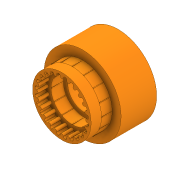
# Autodesk Inventor part: 4th Axis Barrel
Saved by Autodesk Inventor 2020 (Build 240168000, 168)
## iProperties
Created: 2021-06-26
Part Number: 4th Axis Barrel
Material: Generic
Document SubType Name: Modeling
Designer: Coy
Density: 1 g/cm^3
Appearance: Orange
Author: Coy
Autodesk Inventor part; units mm, degrees
ref_plane "YZ Plane" through (0, 0, 0) normal (1, 0, 0) x (0, 1, 0)
ref_plane "XZ Plane" through (0, 0, 0) normal (0, 1, 0) x (-1, 0, 0)
ref_plane "XY Plane" through (0, 0, 0) normal (0, 0, 1) x (1, 0, 0)
sketch "Sketch1" plane through (0, 0, 0) normal (0, 0, 1) x (1, 0, 0)
  circle A0 centre (0, 0) radius 11
  circle A1 centre (0, 0) radius 26
  dimension "d0" = 22
  dimension "d1" = 52
  constraints: 2 centre point, 2 coincident
  measures "d0" diameter of A0
  measures "d1" diameter of A1
extrude "Extrusion1" add sketch "Sketch1" against normal blind 24
sketch "Sketch2" plane through (0, 0, 0) normal (0, 0, 1) x (1, 0, 0)
  circle A0 centre (0, 0) radius 14
  circle A1 centre (0, 0) radius 20
  dimension "d4" = 28
  dimension "d5" = 40
  constraints: 2 centre point, 2 coincident
  measures "d4" diameter of A0
  measures "d5" diameter of A1
extrude "Extrusion2" add sketch "Sketch2" along normal blind 7
chamfer "Chamfer2" distance 7 angle 2 1 edges at (-20, 0, 7) measured on face at (-20, 0, 6.5)
sketch "Sketch4" plane through (0, 0, 7) normal (0, 0, 1) x (1, 0, 0)
  circle A0 centre (0, 0) radius 20 construction
  circle A1 centre (0, 0) radius 19.7556 projected
  arc A2 (0.2, 19.999) -> (-0.2, 19.999) centre (0, 20) ccw
  line L0 (-0.2, 19.999) -> (-0.1988, 19.7546)
  line L1 (0.2, 19.999) -> (0.1988, 19.7546)
  arc A3 (-7.4685, 18.5532) -> (-7.8381, 18.4001) centre (-7.6537, 18.4776) ccw
  line L2 (-7.8381, 18.4001) -> (-7.7434, 18.1748)
  line L3 (-7.4685, 18.5532) -> (-7.3761, 18.3269)
  arc A4 (-14, 14.2828) -> (-14.2828, 14) centre (-14.1421, 14.1421) ccw
  line L4 (-14.2828, 14) -> (-14.1091, 13.828)
  line L5 (-14, 14.2828) -> (-13.828, 14.1091)
  arc A5 (-18.4001, 7.8381) -> (-18.5532, 7.4685) centre (-18.4776, 7.6537) ccw
  line L6 (-18.5532, 7.4685) -> (-18.3269, 7.3761)
  line L7 (-18.4001, 7.8381) -> (-18.1748, 7.7434)
  arc A6 (-19.999, 0.2) -> (-19.999, -0.2) centre (-20, 0) ccw
  line L8 (-19.999, -0.2) -> (-19.7546, -0.1988)
  line L9 (-19.999, 0.2) -> (-19.7546, 0.1988)
  arc A7 (-18.5532, -7.4685) -> (-18.4001, -7.8381) centre (-18.4776, -7.6537) ccw
  line L10 (-18.4001, -7.8381) -> (-18.1748, -7.7434)
  line L11 (-18.5532, -7.4685) -> (-18.3269, -7.3761)
  arc A8 (-14.2828, -14) -> (-14, -14.2828) centre (-14.1421, -14.1421) ccw
  line L12 (-14, -14.2828) -> (-13.828, -14.1091)
  line L13 (-14.2828, -14) -> (-14.1091, -13.828)
  arc A9 (-7.8381, -18.4001) -> (-7.4685, -18.5532) centre (-7.6537, -18.4776) ccw
  line L14 (-7.4685, -18.5532) -> (-7.3761, -18.3269)
  line L15 (-7.8381, -18.4001) -> (-7.7434, -18.1748)
  arc A10 (-0.2, -19.999) -> (0.2, -19.999) centre (0, -20) ccw
  line L16 (0.2, -19.999) -> (0.1988, -19.7546)
  line L17 (-0.2, -19.999) -> (-0.1988, -19.7546)
  arc A11 (7.4685, -18.5532) -> (7.8381, -18.4001) centre (7.6537, -18.4776) ccw
  line L18 (7.8381, -18.4001) -> (7.7434, -18.1748)
  line L19 (7.4685, -18.5532) -> (7.3761, -18.3269)
  arc A12 (14, -14.2828) -> (14.2828, -14) centre (14.1421, -14.1421) ccw
  line L20 (14.2828, -14) -> (14.1091, -13.828)
  line L21 (14, -14.2828) -> (13.828, -14.1091)
  arc A13 (18.4001, -7.8381) -> (18.5532, -7.4685) centre (18.4776, -7.6537) ccw
  line L22 (18.5532, -7.4685) -> (18.3269, -7.3761)
  line L23 (18.4001, -7.8381) -> (18.1748, -7.7434)
  arc A14 (19.999, -0.2) -> (19.999, 0.2) centre (20, 0) ccw
  line L24 (19.999, 0.2) -> (19.7546, 0.1988)
  line L25 (19.999, -0.2) -> (19.7546, -0.1988)
  arc A15 (18.5532, 7.4685) -> (18.4001, 7.8381) centre (18.4776, 7.6537) ccw
  line L26 (18.4001, 7.8381) -> (18.1748, 7.7434)
  line L27 (18.5532, 7.4685) -> (18.3269, 7.3761)
  arc A16 (14.2828, 14) -> (14, 14.2828) centre (14.1421, 14.1421) ccw
  line L28 (14, 14.2828) -> (13.828, 14.1091)
  line L29 (14.2828, 14) -> (14.1091, 13.828)
  arc A17 (7.8381, 18.4001) -> (7.4685, 18.5532) centre (7.6537, 18.4776) ccw
  line L30 (7.4685, 18.5532) -> (7.3761, 18.3269)
  line L31 (7.8381, 18.4001) -> (7.7434, 18.1748)
  dimension "d25" = 0.4
  dimension "d28" = 360
  constraints: 64 end point, 35 point on circle, 16 centre point, 2 tangent, 132 other
  measures "d25" diameter of A2
extrude "Extrusion4" add sketch "Sketch4" against normal up to surface (7 mm away) contours A1 L24 A14 L25 | A1 L26 A15 L27 | L22 A13 L23 A1 | A1 L28 A16 L29 | L20 A12 L21 A1 | A1 L30 A17 L31 | L18 A11 L19 A1 | A1 L0 A2 L1 | L16 A10 L17 A1 | A1 L2 A3 L3 | L14 A9 L15 A1 | A1 L4 A4 L5 | L12 A8 L13 A1 | A1 L6 A5 L7 | L10 A7 L11 A1 | A1 L8 A6 L9
sketch "Sketch8" plane through (0, 0, 0) normal (0, 0, 1) x (1, 0, 0)
  circle A0 centre (0, 0) radius 14 projected
  circle A1 centre (0, 0) radius 11 projected
extrude "Extrusion7" cut sketch "Sketch8" against normal blind 1
chamfer "Chamfer4" distance 8 angle 2 1 edges at (-14, 0, 7) measured on face at (-14, 0, 6.5)
sketch "Sketch10" plane through (0, 0, 7) normal (0, 0, 1) x (1, 0, 0)
  circle A0 centre (0, 0) radius 14 construction
  circle A1 centre (0, 0) radius 14.2794 projected
  arc A2 (-0.2, 13.9986) -> (0.2, 13.9986) centre (0, 14) ccw
  line L0 (0.204, 14.2779) -> (0.2, 13.9971)
  line L1 (-0.204, 14.2779) -> (-0.2, 13.9971)
  line L2 (-7.3156, 12.263) -> (-7.1718, 12.0219)
  arc A3 (-7.1725, 12.0231) -> (-6.8261, 12.2231) centre (-7, 12.1244) ccw
  line L3 (-6.9623, 12.467) -> (-6.8254, 12.2219)
  line L4 (-12.467, 6.9623) -> (-12.2219, 6.8254)
  arc A4 (-12.2231, 6.8261) -> (-12.0231, 7.1725) centre (-12.1244, 7) ccw
  line L5 (-12.263, 7.3156) -> (-12.0219, 7.1718)
  line L6 (-14.2779, -0.204) -> (-13.9971, -0.2)
  arc A5 (-13.9986, -0.2) -> (-13.9986, 0.2) centre (-14, 0) ccw
  line L7 (-14.2779, 0.204) -> (-13.9971, 0.2)
  line L8 (-12.263, -7.3156) -> (-12.0219, -7.1718)
  arc A6 (-12.0231, -7.1725) -> (-12.2231, -6.8261) centre (-12.1244, -7) ccw
  line L9 (-12.467, -6.9623) -> (-12.2219, -6.8254)
  line L10 (-6.9623, -12.467) -> (-6.8254, -12.2219)
  arc A7 (-6.8261, -12.2231) -> (-7.1725, -12.0231) centre (-7, -12.1244) ccw
  line L11 (-7.3156, -12.263) -> (-7.1718, -12.0219)
  line L12 (0.204, -14.2779) -> (0.2, -13.9971)
  arc A8 (0.2, -13.9986) -> (-0.2, -13.9986) centre (0, -14) ccw
  line L13 (-0.204, -14.2779) -> (-0.2, -13.9971)
  line L14 (7.3156, -12.263) -> (7.1718, -12.0219)
  arc A9 (7.1725, -12.0231) -> (6.8261, -12.2231) centre (7, -12.1244) ccw
  line L15 (6.9623, -12.467) -> (6.8254, -12.2219)
  line L16 (12.467, -6.9623) -> (12.2219, -6.8254)
  arc A10 (12.2231, -6.8261) -> (12.0231, -7.1725) centre (12.1244, -7) ccw
  line L17 (12.263, -7.3156) -> (12.0219, -7.1718)
  line L18 (14.2779, 0.204) -> (13.9971, 0.2)
  arc A11 (13.9986, 0.2) -> (13.9986, -0.2) centre (14, 0) ccw
  line L19 (14.2779, -0.204) -> (13.9971, -0.2)
  line L20 (12.263, 7.3156) -> (12.0219, 7.1718)
  arc A12 (12.0231, 7.1725) -> (12.2231, 6.8261) centre (12.1244, 7) ccw
  line L21 (12.467, 6.9623) -> (12.2219, 6.8254)
  line L22 (6.9623, 12.467) -> (6.8254, 12.2219)
  arc A13 (6.8261, 12.2231) -> (7.1725, 12.0231) centre (7, 12.1244) ccw
  line L23 (7.3156, 12.263) -> (7.1718, 12.0219)
  point P0 (13.9986, -0.2)
  point P1 (12.0231, -7.1725)
  point P2 (6.8261, -12.2231)
  point P3 (-0.2, -13.9986)
  point P4 (-7.1725, -12.0231)
  point P5 (7.1725, 12.0231)
  point P6 (0.2, 13.9986)
  point P7 (-12.0231, 7.1725)
  point P8 (-13.9986, 0.2)
  dimension "d67" = 0.4
  dimension "d70" = 360
  constraints: 53 point on circle, 48 end point, 12 centre point, 2 line through centre, 2 tangent, 122 other
  measures "d67" diameter of A2
extrude "Extrusion8" add sketch "Sketch10" against normal up to surface (8 mm away) contours A1 L19 A11 L18 | L21 A12 L20 A1 | A1 L17 A10 L16 | L23 A13 L22 A1 | A1 L15 A9 L14 | L0 A2 L1 A1 | A1 L13 A8 L12 | L3 A3 L2 A1 | A1 L11 A7 L10 | L5 A4 L4 A1 | A1 L9 A6 L8 | L7 A5 L6 A1
sketch "Sketch12" plane through (0, 0, 7) normal (0, 0, 1) x (1, 0, 0)
  circle A0 centre (0, 0) radius 19.7556
  circle A1 centre (0, 0) radius 16.0556 construction
  line L0 (0, 0) -> (0, -27.6947) construction
  arc A2 (1.048, -17.0411) -> (-1.048, -17.0411) centre (0, -17.1056) ccw
  line L1 (-1.0542, -17.1411) -> (-1.048, -17.0411)
  line L2 (1.0542, -17.1411) -> (1.048, -17.0411)
  arc A3 (1.0542, -17.1411) -> (2.2305, -18.1188) centre (2.1022, -17.0766) ccw
  arc A4 (-2.2305, -18.1188) -> (-1.0542, -17.1411) centre (-2.1022, -17.0766) ccw
  arc A5 (5.4547, -16.2842) -> (6.844, -16.9241) centre (6.4503, -15.9507) ccw
  line L3 (5.4547, -16.2842) -> (5.4229, -16.1892)
  arc A6 (5.4229, -16.1892) -> (3.3983, -16.7317) centre (4.4272, -16.5227) ccw
  line L4 (3.4182, -16.8299) -> (3.3983, -16.7317)
  arc A7 (2.535, -18.0787) -> (3.4182, -16.8299) centre (2.3892, -17.0389) ccw
  arc A8 (9.4835, -14.3175) -> (10.991, -14.5761) centre (10.3589, -13.7377) ccw
  line L5 (9.4835, -14.3175) -> (9.4282, -14.234)
  arc A9 (9.4282, -14.234) -> (7.6129, -15.282) centre (8.5528, -14.8138) ccw
  line L6 (7.6576, -15.3717) -> (7.6129, -15.282)
  arc A10 (7.1277, -16.8066) -> (7.6576, -15.3717) centre (6.7178, -15.8399) ccw
  arc A11 (12.866, -11.3752) -> (14.3891, -11.2347) centre (13.5615, -10.5885) ccw
  line L7 (12.866, -11.3752) -> (12.7909, -11.3088)
  arc A12 (12.7909, -11.3088) -> (11.3088, -12.7909) centre (12.0955, -12.0955) ccw
  line L8 (11.3752, -12.866) -> (11.3088, -12.7909)
  arc A13 (11.2347, -14.3891) -> (11.3752, -12.866) centre (10.5885, -13.5615) ccw
  arc A14 (15.3717, -7.6576) -> (16.8066, -7.1277) centre (15.8399, -6.7178) ccw
  line L9 (15.3717, -7.6576) -> (15.282, -7.6129)
  arc A15 (15.282, -7.6129) -> (14.234, -9.4282) centre (14.8138, -8.5528) ccw
  line L10 (14.3175, -9.4835) -> (14.234, -9.4282)
  arc A16 (14.5761, -10.991) -> (14.3175, -9.4835) centre (13.7377, -10.3589) ccw
  arc A17 (16.8299, -3.4182) -> (18.0787, -2.535) centre (17.0389, -2.3892) ccw
  line L11 (16.8299, -3.4182) -> (16.7317, -3.3983)
  arc A18 (16.7317, -3.3983) -> (16.1892, -5.4229) centre (16.5227, -4.4272) ccw
  line L12 (16.2842, -5.4547) -> (16.1892, -5.4229)
  arc A19 (16.9241, -6.844) -> (16.2842, -5.4547) centre (15.9507, -6.4503) ccw
  arc A20 (17.1411, 1.0542) -> (18.1188, 2.2305) centre (17.0766, 2.1022) ccw
  line L13 (17.1411, 1.0542) -> (17.0411, 1.048)
  arc A21 (17.0411, 1.048) -> (17.0411, -1.048) centre (17.1056, 0) ccw
  line L14 (17.1411, -1.0542) -> (17.0411, -1.048)
  arc A22 (18.1188, -2.2305) -> (17.1411, -1.0542) centre (17.0766, -2.1022) ccw
  arc A23 (16.2842, 5.4547) -> (16.9241, 6.844) centre (15.9507, 6.4503) ccw
  line L15 (16.2842, 5.4547) -> (16.1892, 5.4229)
  arc A24 (16.1892, 5.4229) -> (16.7317, 3.3983) centre (16.5227, 4.4272) ccw
  line L16 (16.8299, 3.4182) -> (16.7317, 3.3983)
  arc A25 (18.0787, 2.535) -> (16.8299, 3.4182) centre (17.0389, 2.3892) ccw
  arc A26 (14.3175, 9.4835) -> (14.5761, 10.991) centre (13.7377, 10.3589) ccw
  line L17 (14.3175, 9.4835) -> (14.234, 9.4282)
  arc A27 (14.234, 9.4282) -> (15.282, 7.6129) centre (14.8138, 8.5528) ccw
  line L18 (15.3717, 7.6576) -> (15.282, 7.6129)
  arc A28 (16.8066, 7.1277) -> (15.3717, 7.6576) centre (15.8399, 6.7178) ccw
  arc A29 (11.3752, 12.866) -> (11.2347, 14.3891) centre (10.5885, 13.5615) ccw
  line L19 (11.3752, 12.866) -> (11.3088, 12.7909)
  arc A30 (11.3088, 12.7909) -> (12.7909, 11.3088) centre (12.0955, 12.0955) ccw
  line L20 (12.866, 11.3752) -> (12.7909, 11.3088)
  arc A31 (14.3891, 11.2347) -> (12.866, 11.3752) centre (13.5615, 10.5885) ccw
  arc A32 (7.6576, 15.3717) -> (7.1277, 16.8066) centre (6.7178, 15.8399) ccw
  line L21 (7.6576, 15.3717) -> (7.6129, 15.282)
  arc A33 (7.6129, 15.282) -> (9.4282, 14.234) centre (8.5528, 14.8138) ccw
  line L22 (9.4835, 14.3175) -> (9.4282, 14.234)
  arc A34 (10.991, 14.5761) -> (9.4835, 14.3175) centre (10.3589, 13.7377) ccw
  arc A35 (3.4182, 16.8299) -> (2.535, 18.0787) centre (2.3892, 17.0389) ccw
  line L23 (3.4182, 16.8299) -> (3.3983, 16.7317)
  arc A36 (3.3983, 16.7317) -> (5.4229, 16.1892) centre (4.4272, 16.5227) ccw
  line L24 (5.4547, 16.2842) -> (5.4229, 16.1892)
  arc A37 (6.844, 16.9241) -> (5.4547, 16.2842) centre (6.4503, 15.9507) ccw
  arc A38 (-1.0542, 17.1411) -> (-2.2305, 18.1188) centre (-2.1022, 17.0766) ccw
  line L25 (-1.0542, 17.1411) -> (-1.048, 17.0411)
  arc A39 (-1.048, 17.0411) -> (1.048, 17.0411) centre (0, 17.1056) ccw
  line L26 (1.0542, 17.1411) -> (1.048, 17.0411)
  arc A40 (2.2305, 18.1188) -> (1.0542, 17.1411) centre (2.1022, 17.0766) ccw
  arc A41 (-5.4547, 16.2842) -> (-6.844, 16.9241) centre (-6.4503, 15.9507) ccw
  line L27 (-5.4547, 16.2842) -> (-5.4229, 16.1892)
  arc A42 (-5.4229, 16.1892) -> (-3.3983, 16.7317) centre (-4.4272, 16.5227) ccw
  line L28 (-3.4182, 16.8299) -> (-3.3983, 16.7317)
  arc A43 (-2.535, 18.0787) -> (-3.4182, 16.8299) centre (-2.3892, 17.0389) ccw
  arc A44 (-9.4835, 14.3175) -> (-10.991, 14.5761) centre (-10.3589, 13.7377) ccw
  line L29 (-9.4835, 14.3175) -> (-9.4282, 14.234)
  arc A45 (-9.4282, 14.234) -> (-7.6129, 15.282) centre (-8.5528, 14.8138) ccw
  line L30 (-7.6576, 15.3717) -> (-7.6129, 15.282)
  arc A46 (-7.1277, 16.8066) -> (-7.6576, 15.3717) centre (-6.7178, 15.8399) ccw
  arc A47 (-12.866, 11.3752) -> (-14.3891, 11.2347) centre (-13.5615, 10.5885) ccw
  line L31 (-12.866, 11.3752) -> (-12.7909, 11.3088)
  arc A48 (-12.7909, 11.3088) -> (-11.3088, 12.7909) centre (-12.0955, 12.0955) ccw
  line L32 (-11.3752, 12.866) -> (-11.3088, 12.7909)
  arc A49 (-11.2347, 14.3891) -> (-11.3752, 12.866) centre (-10.5885, 13.5615) ccw
  arc A50 (-15.3717, 7.6576) -> (-16.8066, 7.1277) centre (-15.8399, 6.7178) ccw
  line L33 (-15.3717, 7.6576) -> (-15.282, 7.6129)
  arc A51 (-15.282, 7.6129) -> (-14.234, 9.4282) centre (-14.8138, 8.5528) ccw
  line L34 (-14.3175, 9.4835) -> (-14.234, 9.4282)
  arc A52 (-14.5761, 10.991) -> (-14.3175, 9.4835) centre (-13.7377, 10.3589) ccw
  arc A53 (-16.8299, 3.4182) -> (-18.0787, 2.535) centre (-17.0389, 2.3892) ccw
  line L35 (-16.8299, 3.4182) -> (-16.7317, 3.3983)
  arc A54 (-16.7317, 3.3983) -> (-16.1892, 5.4229) centre (-16.5227, 4.4272) ccw
  line L36 (-16.2842, 5.4547) -> (-16.1892, 5.4229)
  arc A55 (-16.9241, 6.844) -> (-16.2842, 5.4547) centre (-15.9507, 6.4503) ccw
  arc A56 (-17.1411, -1.0542) -> (-18.1188, -2.2305) centre (-17.0766, -2.1022) ccw
  line L37 (-17.1411, -1.0542) -> (-17.0411, -1.048)
  arc A57 (-17.0411, -1.048) -> (-17.0411, 1.048) centre (-17.1056, 0) ccw
  line L38 (-17.1411, 1.0542) -> (-17.0411, 1.048)
  arc A58 (-18.1188, 2.2305) -> (-17.1411, 1.0542) centre (-17.0766, 2.1022) ccw
  arc A59 (-16.2842, -5.4547) -> (-16.9241, -6.844) centre (-15.9507, -6.4503) ccw
  line L39 (-16.2842, -5.4547) -> (-16.1892, -5.4229)
  arc A60 (-16.1892, -5.4229) -> (-16.7317, -3.3983) centre (-16.5227, -4.4272) ccw
  line L40 (-16.8299, -3.4182) -> (-16.7317, -3.3983)
  arc A61 (-18.0787, -2.535) -> (-16.8299, -3.4182) centre (-17.0389, -2.3892) ccw
  arc A62 (-14.3175, -9.4835) -> (-14.5761, -10.991) centre (-13.7377, -10.3589) ccw
  line L41 (-14.3175, -9.4835) -> (-14.234, -9.4282)
  arc A63 (-14.234, -9.4282) -> (-15.282, -7.6129) centre (-14.8138, -8.5528) ccw
  line L42 (-15.3717, -7.6576) -> (-15.282, -7.6129)
  arc A64 (-16.8066, -7.1277) -> (-15.3717, -7.6576) centre (-15.8399, -6.7178) ccw
  arc A65 (-11.3752, -12.866) -> (-11.2347, -14.3891) centre (-10.5885, -13.5615) ccw
  line L43 (-11.3752, -12.866) -> (-11.3088, -12.7909)
  arc A66 (-11.3088, -12.7909) -> (-12.7909, -11.3088) centre (-12.0955, -12.0955) ccw
  line L44 (-12.866, -11.3752) -> (-12.7909, -11.3088)
  arc A67 (-14.3891, -11.2347) -> (-12.866, -11.3752) centre (-13.5615, -10.5885) ccw
  arc A68 (-7.6576, -15.3717) -> (-7.1277, -16.8066) centre (-6.7178, -15.8399) ccw
  line L45 (-7.6576, -15.3717) -> (-7.6129, -15.282)
  arc A69 (-7.6129, -15.282) -> (-9.4282, -14.234) centre (-8.5528, -14.8138) ccw
  line L46 (-9.4835, -14.3175) -> (-9.4282, -14.234)
  arc A70 (-10.991, -14.5761) -> (-9.4835, -14.3175) centre (-10.3589, -13.7377) ccw
  arc A71 (-3.4182, -16.8299) -> (-2.535, -18.0787) centre (-2.3892, -17.0389) ccw
  line L47 (-3.4182, -16.8299) -> (-3.3983, -16.7317)
  arc A72 (-3.3983, -16.7317) -> (-5.4229, -16.1892) centre (-4.4272, -16.5227) ccw
  line L48 (-5.4547, -16.2842) -> (-5.4229, -16.1892)
  arc A73 (-6.844, -16.9241) -> (-5.4547, -16.2842) centre (-6.4503, -15.9507) ccw
  arc A74 (2.2305, -18.1188) -> (2.535, -18.0787) centre (0, 0) ccw
  arc A75 (6.844, -16.9241) -> (7.1277, -16.8066) centre (0, 0) ccw
  arc A76 (10.991, -14.5761) -> (11.2347, -14.3891) centre (0, 0) ccw
  arc A77 (14.3891, -11.2347) -> (14.5761, -10.991) centre (0, 0) ccw
  arc A78 (16.8066, -7.1277) -> (16.9241, -6.844) centre (0, 0) ccw
  arc A79 (18.0787, -2.535) -> (18.1188, -2.2305) centre (0, 0) ccw
  arc A80 (18.1188, 2.2305) -> (18.0787, 2.535) centre (0, 0) ccw
  arc A81 (16.9241, 6.844) -> (16.8066, 7.1277) centre (0, 0) ccw
  arc A82 (14.5761, 10.991) -> (14.3891, 11.2347) centre (0, 0) ccw
  arc A83 (11.2347, 14.3891) -> (10.991, 14.5761) centre (0, 0) ccw
  arc A84 (7.1277, 16.8066) -> (6.844, 16.9241) centre (0, 0) ccw
  arc A85 (2.535, 18.0787) -> (2.2305, 18.1188) centre (0, 0) ccw
  arc A86 (-2.2305, 18.1188) -> (-2.535, 18.0787) centre (0, 0) ccw
  arc A87 (-6.844, 16.9241) -> (-7.1277, 16.8066) centre (0, 0) ccw
  arc A88 (-10.991, 14.5761) -> (-11.2347, 14.3891) centre (0, 0) ccw
  arc A89 (-14.3891, 11.2347) -> (-14.5761, 10.991) centre (0, 0) ccw
  arc A90 (-16.8066, 7.1277) -> (-16.9241, 6.844) centre (0, 0) ccw
  arc A91 (-18.0787, 2.535) -> (-18.1188, 2.2305) centre (0, 0) ccw
  arc A92 (-18.1188, -2.2305) -> (-18.0787, -2.535) centre (0, 0) ccw
  arc A93 (-16.9241, -6.844) -> (-16.8066, -7.1277) centre (0, 0) ccw
  arc A94 (-14.5761, -10.991) -> (-14.3891, -11.2347) centre (0, 0) ccw
  arc A95 (-11.2347, -14.3891) -> (-10.991, -14.5761) centre (0, 0) ccw
  arc A96 (-7.1277, -16.8066) -> (-6.844, -16.9241) centre (0, 0) ccw
  arc A97 (-2.535, -18.0787) -> (-2.2305, -18.1188) centre (0, 0) ccw
  dimension "d85" = 2.1
  dimension "d86" = 2.1
  dimension "d87" = 2.1
  dimension "d90" = 360
  constraints: 144 point on circle, 96 end point, 72 centre point, 4 tangent, 1 vertical alignment, 464 other
  measures "d85" diameter of A2
  measures "d86" diameter of A4
  measures "d87" diameter of A3
ref_plane "Work Plane1" through (0, 0, 14) normal (0, 0, 1) x (1, 0, 0)
sketch "Sketch13" plane through (0, 0, 14) normal (0, 0, 1) x (1, 0, 0)
  circle A0 centre (0, 0) radius 19.7556
  circle A1 centre (0, 0) radius 16.0556 construction
  line L0 (0, 0) -> (0.8023, -27.6831) construction
  arc A2 (1.5412, -17.0036) -> (-0.5539, -17.0643) centre (0.4955, -17.0984) ccw
  line L1 (-0.5572, -17.1644) -> (-0.5539, -17.0643)
  line L2 (1.5503, -17.1034) -> (1.5412, -17.0036)
  arc A3 (1.5503, -17.1034) -> (2.7544, -18.0466) centre (2.596, -17.0086) ccw
  arc A4 (-1.7047, -18.1758) -> (-0.5572, -17.1644) centre (-1.6066, -17.1304) ccw
  arc A5 (5.9241, -16.1193) -> (7.3314, -16.7187) centre (6.9097, -15.7571) ccw
  line L3 (5.9241, -16.1193) -> (5.8896, -16.0253)
  arc A6 (5.8896, -16.0253) -> (3.8815, -16.6262) centre (4.904, -16.3875) ccw
  line L4 (3.9043, -16.7238) -> (3.8815, -16.6262)
  arc A7 (3.0577, -17.9977) -> (3.9043, -16.7238) centre (2.8818, -16.9625) ccw
  arc A8 (9.8943, -14.0368) -> (11.4087, -14.2516) centre (10.7525, -13.4319) ccw
  line L5 (9.8943, -14.0368) -> (9.8365, -13.9549)
  arc A9 (9.8365, -13.9549) -> (8.0524, -15.0551) centre (8.9783, -14.5599) ccw
  line L6 (8.0997, -15.1434) -> (8.0524, -15.0551)
  arc A10 (7.6116, -16.593) -> (8.0997, -15.1434) centre (7.1738, -15.6387) ccw
  arc A11 (13.1901, -10.9977) -> (14.7085, -10.8132) centre (13.8625, -10.1912) ccw
  line L7 (13.1901, -10.9977) -> (13.1132, -10.9335)
  arc A12 (13.1132, -10.9335) -> (11.6746, -12.458) centre (12.4408, -11.74) ccw
  line L8 (11.7431, -12.5311) -> (11.6746, -12.458)
  arc A13 (11.6468, -14.0576) -> (11.7431, -12.5311) centre (10.977, -13.2491) ccw
  arc A14 (15.5871, -7.2091) -> (17.006, -6.6379) centre (16.0279, -6.2561) ccw
  line L9 (15.5871, -7.2091) -> (15.4962, -7.167)
  arc A15 (15.4962, -7.167) -> (14.5012, -9.0119) centre (15.0554, -8.1201) ccw
  line L10 (14.5863, -9.0648) -> (14.5012, -9.0119)
  arc A16 (14.8884, -10.5642) -> (14.5863, -9.0648) centre (14.032, -9.9566) ccw
  arc A17 (16.9218, -2.9292) -> (18.1445, -2.0102) centre (17.1009, -1.8946) ccw
  line L11 (16.9218, -2.9292) -> (16.8231, -2.9121)
  arc A18 (16.8231, -2.9121) -> (16.3395, -4.9516) centre (16.644, -3.9467) ccw
  line L12 (16.4354, -4.9807) -> (16.3395, -4.9516)
  arc A19 (17.1153, -6.3508) -> (16.4354, -4.9807) centre (16.1309, -5.9855) ccw
  arc A20 (17.1034, 1.5503) -> (18.0466, 2.7544) centre (17.0086, 2.596) ccw
  line L13 (17.1034, 1.5503) -> (17.0036, 1.5412)
  arc A21 (17.0036, 1.5412) -> (17.0643, -0.5539) centre (17.0984, 0.4955) ccw
  line L14 (17.1644, -0.5572) -> (17.0643, -0.5539)
  arc A22 (18.1758, -1.7047) -> (17.1644, -0.5572) centre (17.1304, -1.6066) ccw
  arc A23 (16.1193, 5.9241) -> (16.7187, 7.3314) centre (15.7571, 6.9097) ccw
  line L15 (16.1193, 5.9241) -> (16.0253, 5.8896)
  arc A24 (16.0253, 5.8896) -> (16.6262, 3.8815) centre (16.3875, 4.904) ccw
  line L16 (16.7238, 3.9043) -> (16.6262, 3.8815)
  arc A25 (17.9977, 3.0577) -> (16.7238, 3.9043) centre (16.9625, 2.8818) ccw
  arc A26 (14.0368, 9.8943) -> (14.2516, 11.4087) centre (13.4319, 10.7525) ccw
  line L17 (14.0368, 9.8943) -> (13.9549, 9.8365)
  arc A27 (13.9549, 9.8365) -> (15.0551, 8.0524) centre (14.5599, 8.9783) ccw
  line L18 (15.1434, 8.0997) -> (15.0551, 8.0524)
  arc A28 (16.593, 7.6116) -> (15.1434, 8.0997) centre (15.6387, 7.1738) ccw
  arc A29 (10.9977, 13.1901) -> (10.8132, 14.7085) centre (10.1912, 13.8625) ccw
  line L19 (10.9977, 13.1901) -> (10.9335, 13.1132)
  arc A30 (10.9335, 13.1132) -> (12.458, 11.6746) centre (11.74, 12.4408) ccw
  line L20 (12.5311, 11.7431) -> (12.458, 11.6746)
  arc A31 (14.0576, 11.6468) -> (12.5311, 11.7431) centre (13.2491, 10.977) ccw
  arc A32 (7.2091, 15.5871) -> (6.6379, 17.006) centre (6.2561, 16.0279) ccw
  line L21 (7.2091, 15.5871) -> (7.167, 15.4962)
  arc A33 (7.167, 15.4962) -> (9.0119, 14.5012) centre (8.1201, 15.0554) ccw
  line L22 (9.0648, 14.5863) -> (9.0119, 14.5012)
  arc A34 (10.5642, 14.8884) -> (9.0648, 14.5863) centre (9.9566, 14.032) ccw
  arc A35 (2.9292, 16.9218) -> (2.0102, 18.1445) centre (1.8946, 17.1009) ccw
  line L23 (2.9292, 16.9218) -> (2.9121, 16.8231)
  arc A36 (2.9121, 16.8231) -> (4.9516, 16.3395) centre (3.9467, 16.644) ccw
  line L24 (4.9807, 16.4354) -> (4.9516, 16.3395)
  arc A37 (6.3508, 17.1153) -> (4.9807, 16.4354) centre (5.9855, 16.1309) ccw
  arc A38 (-1.5503, 17.1034) -> (-2.7544, 18.0466) centre (-2.596, 17.0086) ccw
  line L25 (-1.5503, 17.1034) -> (-1.5412, 17.0036)
  arc A39 (-1.5412, 17.0036) -> (0.5539, 17.0643) centre (-0.4955, 17.0984) ccw
  line L26 (0.5572, 17.1644) -> (0.5539, 17.0643)
  arc A40 (1.7047, 18.1758) -> (0.5572, 17.1644) centre (1.6066, 17.1304) ccw
  arc A41 (-5.9241, 16.1193) -> (-7.3314, 16.7187) centre (-6.9097, 15.7571) ccw
  line L27 (-5.9241, 16.1193) -> (-5.8896, 16.0253)
  arc A42 (-5.8896, 16.0253) -> (-3.8815, 16.6262) centre (-4.904, 16.3875) ccw
  line L28 (-3.9043, 16.7238) -> (-3.8815, 16.6262)
  arc A43 (-3.0577, 17.9977) -> (-3.9043, 16.7238) centre (-2.8818, 16.9625) ccw
  arc A44 (-9.8943, 14.0368) -> (-11.4087, 14.2516) centre (-10.7525, 13.4319) ccw
  line L29 (-9.8943, 14.0368) -> (-9.8365, 13.9549)
  arc A45 (-9.8365, 13.9549) -> (-8.0524, 15.0551) centre (-8.9783, 14.5599) ccw
  line L30 (-8.0997, 15.1434) -> (-8.0524, 15.0551)
  arc A46 (-7.6116, 16.593) -> (-8.0997, 15.1434) centre (-7.1738, 15.6387) ccw
  arc A47 (-13.1901, 10.9977) -> (-14.7085, 10.8132) centre (-13.8625, 10.1912) ccw
  line L31 (-13.1901, 10.9977) -> (-13.1132, 10.9335)
  arc A48 (-13.1132, 10.9335) -> (-11.6746, 12.458) centre (-12.4408, 11.74) ccw
  line L32 (-11.7431, 12.5311) -> (-11.6746, 12.458)
  arc A49 (-11.6468, 14.0576) -> (-11.7431, 12.5311) centre (-10.977, 13.2491) ccw
  arc A50 (-15.5871, 7.2091) -> (-17.006, 6.6379) centre (-16.0279, 6.2561) ccw
  line L33 (-15.5871, 7.2091) -> (-15.4962, 7.167)
  arc A51 (-15.4962, 7.167) -> (-14.5012, 9.0119) centre (-15.0554, 8.1201) ccw
  line L34 (-14.5863, 9.0648) -> (-14.5012, 9.0119)
  arc A52 (-14.8884, 10.5642) -> (-14.5863, 9.0648) centre (-14.032, 9.9566) ccw
  arc A53 (-16.9218, 2.9292) -> (-18.1445, 2.0102) centre (-17.1009, 1.8946) ccw
  line L35 (-16.9218, 2.9292) -> (-16.8231, 2.9121)
  arc A54 (-16.8231, 2.9121) -> (-16.3395, 4.9516) centre (-16.644, 3.9467) ccw
  line L36 (-16.4354, 4.9807) -> (-16.3395, 4.9516)
  arc A55 (-17.1153, 6.3508) -> (-16.4354, 4.9807) centre (-16.1309, 5.9855) ccw
  arc A56 (-17.1034, -1.5503) -> (-18.0466, -2.7544) centre (-17.0086, -2.596) ccw
  line L37 (-17.1034, -1.5503) -> (-17.0036, -1.5412)
  arc A57 (-17.0036, -1.5412) -> (-17.0643, 0.5539) centre (-17.0984, -0.4955) ccw
  line L38 (-17.1644, 0.5572) -> (-17.0643, 0.5539)
  arc A58 (-18.1758, 1.7047) -> (-17.1644, 0.5572) centre (-17.1304, 1.6066) ccw
  arc A59 (-16.1193, -5.9241) -> (-16.7187, -7.3314) centre (-15.7571, -6.9097) ccw
  line L39 (-16.1193, -5.9241) -> (-16.0253, -5.8896)
  arc A60 (-16.0253, -5.8896) -> (-16.6262, -3.8815) centre (-16.3875, -4.904) ccw
  line L40 (-16.7238, -3.9043) -> (-16.6262, -3.8815)
  arc A61 (-17.9977, -3.0577) -> (-16.7238, -3.9043) centre (-16.9625, -2.8818) ccw
  arc A62 (-14.0368, -9.8943) -> (-14.2516, -11.4087) centre (-13.4319, -10.7525) ccw
  line L41 (-14.0368, -9.8943) -> (-13.9549, -9.8365)
  arc A63 (-13.9549, -9.8365) -> (-15.0551, -8.0524) centre (-14.5599, -8.9783) ccw
  line L42 (-15.1434, -8.0997) -> (-15.0551, -8.0524)
  arc A64 (-16.593, -7.6116) -> (-15.1434, -8.0997) centre (-15.6387, -7.1738) ccw
  arc A65 (-10.9977, -13.1901) -> (-10.8132, -14.7085) centre (-10.1912, -13.8625) ccw
  line L43 (-10.9977, -13.1901) -> (-10.9335, -13.1132)
  arc A66 (-10.9335, -13.1132) -> (-12.458, -11.6746) centre (-11.74, -12.4408) ccw
  line L44 (-12.5311, -11.7431) -> (-12.458, -11.6746)
  arc A67 (-14.0576, -11.6468) -> (-12.5311, -11.7431) centre (-13.2491, -10.977) ccw
  arc A68 (-7.2091, -15.5871) -> (-6.6379, -17.006) centre (-6.2561, -16.0279) ccw
  line L45 (-7.2091, -15.5871) -> (-7.167, -15.4962)
  arc A69 (-7.167, -15.4962) -> (-9.0119, -14.5012) centre (-8.1201, -15.0554) ccw
  line L46 (-9.0648, -14.5863) -> (-9.0119, -14.5012)
  arc A70 (-10.5642, -14.8884) -> (-9.0648, -14.5863) centre (-9.9566, -14.032) ccw
  arc A71 (-2.9292, -16.9218) -> (-2.0102, -18.1445) centre (-1.8946, -17.1009) ccw
  line L47 (-2.9292, -16.9218) -> (-2.9121, -16.8231)
  arc A72 (-2.9121, -16.8231) -> (-4.9516, -16.3395) centre (-3.9467, -16.644) ccw
  line L48 (-4.9807, -16.4354) -> (-4.9516, -16.3395)
  arc A73 (-6.3508, -17.1153) -> (-4.9807, -16.4354) centre (-5.9855, -16.1309) ccw
  arc A74 (2.7544, -18.0466) -> (3.0577, -17.9977) centre (0, 0) ccw
  arc A75 (7.3314, -16.7187) -> (7.6116, -16.593) centre (0, 0) ccw
  arc A76 (11.4087, -14.2516) -> (11.6468, -14.0576) centre (0, 0) ccw
  arc A77 (14.7085, -10.8132) -> (14.8884, -10.5642) centre (0, 0) ccw
  arc A78 (17.006, -6.6379) -> (17.1153, -6.3508) centre (0, 0) ccw
  arc A79 (18.1445, -2.0102) -> (18.1758, -1.7047) centre (0, 0) ccw
  arc A80 (18.0466, 2.7544) -> (17.9977, 3.0577) centre (0, 0) ccw
  arc A81 (16.7187, 7.3314) -> (16.593, 7.6116) centre (0, 0) ccw
  arc A82 (14.2516, 11.4087) -> (14.0576, 11.6468) centre (0, 0) ccw
  arc A83 (10.8132, 14.7085) -> (10.5642, 14.8884) centre (0, 0) ccw
  arc A84 (6.6379, 17.006) -> (6.3508, 17.1153) centre (0, 0) ccw
  arc A85 (2.0102, 18.1445) -> (1.7047, 18.1758) centre (0, 0) ccw
  arc A86 (-2.7544, 18.0466) -> (-3.0577, 17.9977) centre (0, 0) ccw
  arc A87 (-7.3314, 16.7187) -> (-7.6116, 16.593) centre (0, 0) ccw
  arc A88 (-11.4087, 14.2516) -> (-11.6468, 14.0576) centre (0, 0) ccw
  arc A89 (-14.7085, 10.8132) -> (-14.8884, 10.5642) centre (0, 0) ccw
  arc A90 (-17.006, 6.6379) -> (-17.1153, 6.3508) centre (0, 0) ccw
  arc A91 (-18.1445, 2.0102) -> (-18.1758, 1.7047) centre (0, 0) ccw
  arc A92 (-18.0466, -2.7544) -> (-17.9977, -3.0577) centre (0, 0) ccw
  arc A93 (-16.7187, -7.3314) -> (-16.593, -7.6116) centre (0, 0) ccw
  arc A94 (-14.2516, -11.4087) -> (-14.0576, -11.6468) centre (0, 0) ccw
  arc A95 (-10.8132, -14.7085) -> (-10.5642, -14.8884) centre (0, 0) ccw
  arc A96 (-6.6379, -17.006) -> (-6.3508, -17.1153) centre (0, 0) ccw
  arc A97 (-2.0102, -18.1445) -> (-1.7047, -18.1758) centre (0, 0) ccw
  point P0 (0, 0)
  dimension "d95" = 2.1
  dimension "d96" = 2.1
  dimension "d97" = 2.1
  dimension "d98" = 360
  constraints: 144 point on circle, 96 end point, 72 centre point, 4 tangent, 465 other
  measures "d95" diameter of A2
  measures "d96" diameter of A4
  measures "d97" diameter of A3
extrude "Extrusion10" add sketch "Sketch12" along normal blind 7
equation "\"d86\" = d85"
equation "\"d87\" = d85"
equation "\"d96\" = d95"
equation "\"d97\" = d95"
body "Solid1"
